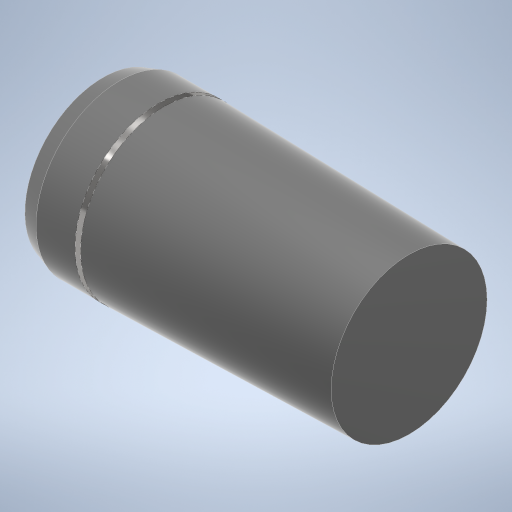
# Autodesk Inventor part: 3.2MEGA-PIXELS-WEBCAMERA
Saved by Autodesk Inventor 2024.1 (Build 281209000, 209)
## iProperties
Created: 2024-02-13
Part Number: 3.2MEGA-PIXELS-WEBCAMERA
Material: アルミニウム 6061
Document SubType Name: Modeling
Designer: haruy
Density: 2.7 g/cm^3
Appearance: アルミニウム - フラット
Author: haruy
Autodesk Inventor part; units mm, degrees
sketch "スケッチ1" plane through (0, 0, 0) normal (1, 0, 0) x (0, 1, 0)
  circle A0 centre (0, 0) radius 15
  point P0 (15, 0)
  dimension "d0" = 30
  constraints: 1 coincident, 1 horizontal alignment, 2 other
ref_plane "作業平面1" through (52, 0, 0) normal (1, 0, 0) x (0, 1, 0)
sketch "スケッチ2" plane through (52, 0, 0) normal (1, 0, 0) x (0, 1, 0)
  circle A0 centre (0, 0) radius 14
  line L0 (-12.3996, 6.5) -> (-12.3996, -6.5)
  dimension "d2" = 28
  dimension "d36" = 13
  constraints: 2 end point, 2 point on circle, 1 centre point, 1 coincident, 1 vertical
  measures "d2" diameter of A0
  measures "d36" distance of L0.start L0.end
ref_plane "作業平面2" through (-3, 0, 0) normal (1, 0, 0) x (0, 1, 0)
sketch "スケッチ3" plane through (-3, 0, 0) normal (1, 0, 0) x (0, 1, 0)
  circle A0 centre (0, 0) radius 14
  dimension "d4" = 28
  constraints: 1 centre point, 1 coincident
  measures "d4" diameter of A0
ref_plane "作業平面3" through (0, 0, 0) normal (0, 0, -1) x (0, 1, 0)
ref_plane "作業平面5" through (8, 0, 0) normal (1, 0, 0) x (0, 1, 0)
ref_plane "作業平面4" through (7, 0, 0) normal (1, 0, 0) x (0, 1, 0)
sketch "スケッチ5" plane through (7, 0, 0) normal (1, 0, 0) x (0, 1, 0)
  circle A0 centre (0, 0) radius 15
  dimension "d20" = 30
  constraints: 1 centre point, 1 coincident
  measures "d20" diameter of A0
sketch "スケッチ6" plane through (8, 0, 0) normal (1, 0, 0) x (0, 1, 0)
  circle A0 centre (0, 0) radius 15
  dimension "d21" = 30
  constraints: 1 centre point, 1 coincident
  measures "d21" diameter of A0
loft "ロフト3" add profiles "スケッチ5", "スケッチ6"
extrude "押し出し1" add sketch "スケッチ1" along normal up to surface (7 mm away) separate body
loft "ロフト4" add profiles "スケッチ3" bodies 2 section 2 edges at (0, -15, 0)
loft "ロフト5" add profiles "スケッチ2" separate body section 2 edges at (8, -15, 0)
